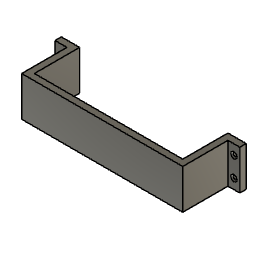
Bracket 185x155x50mm (Autodesk Fusion 360 design; units mm, degrees)
Autodesk Fusion 360 part; units mm, degrees
sketch "Outline" plane through (0, 0, 0) normal (0, 0, 1) x (1, 0, 0)
  line L0 (0, 0) -> (0, 56.9537) construction
  line L1 (0, 0) -> (93.5, 0)
  line L2 (93.5, 0) -> (93.5, 57)
  line L3 (93.5, 57) -> (116.5, 57)
  line L4 (116.5, 57) -> (116.5, 49)
  line L5 (-93.5, 57) -> (-116.5, 57)
  line L6 (-93.5, 0) -> (-93.5, 57)
  line L7 (0, 0) -> (-93.5, 0)
  line L8 (-101.5, -8) -> (-101.5, 49)
  line L9 (-101.5, 49) -> (-116.5, 49)
  line L10 (-116.5, 57) -> (-116.5, 49)
  line L11 (101.5, -8) -> (101.5, 49)
  line L12 (101.5, 49) -> (116.5, 49)
  line L13 (-101.5, -8) -> (101.5, -8)
  dimension "d2" = 187
  dimension "d3" = 57
  dimension "d6" = 23
  dimension "d8" = 8
  dimension "d9" = 8
  dimension "d10" = 8
  constraint coincident L0.start L1.start
  constraint vertical L0
  constraint perpendicular L0 L1
  constraint perpendicular L1 L2
  constraint perpendicular L2 L3
  constraint symmetric L0 L1.start L7.start
  constraint symmetric L0 L1.end L6.start
  constraint symmetric L0 L2.end L5.start
  constraint symmetric L0 L3.end L5.end
  constraint parallel L7 L13
  constraint vertical L8
  constraint horizontal L9
  constraint vertical L4
  constraint vertical L10
  measures "d2" distance of L1.end L6.start
  measures "d3" distance of L1.end L2.end
  measures "d6" distance of L5.start L5.end
  measures "d8" distance of L6 L8
  measures "d9" distance of L5 L9
  measures "d10" distance of L7 L13
extrude "Extrude1" add sketch "Outline" along normal blind 50
sketch "Holes for Mounting" plane through (0, 49, 0) normal (0, -1, 0) x (1, 0, 0)
  line L0 (-116.5, 0) -> (-101.5, 0)
  line L1 (-101.5, 0) -> (-101.5, 50)
  line L2 (-101.5, 50) -> (-116.5, 50)
  line L3 (-116.5, 50) -> (-116.5, 0)
  line L4 (101.5, 0) -> (116.5, 0)
  line L5 (116.5, 0) -> (116.5, 50)
  line L6 (116.5, 50) -> (101.5, 50)
  line L7 (101.5, 50) -> (101.5, 0)
  line L8 (0, 0) -> (0, 29.5518) construction
  line L9 (-109, 50) -> (-109, 0) construction
  circle A0 centre (-109, 12.5) radius 4
  line L10 (-116.5, 25) -> (-101.5, 25) construction
  circle A1 centre (-109, 37.5) radius 4
  circle A2 centre (109, 12.5) radius 4
  circle A3 centre (109, 37.5) radius 4
  dimension "d13" = 25
  dimension "d14" = 8
  constraint coincident L8.start origin
  constraint vertical L8
  constraint midpoint L2 L9.start
  constraint midpoint L0 L9.end
  constraint coincident L9 A0.centre
  constraint midpoint L3 L10.start
  constraint midpoint L1 L10.end
  constraint symmetric A0 L10 A1
  constraint symmetric L8 A0 A2
  constraint symmetric L8 A1 A3
  measures "d13" distance of A0.centre A1.centre
  measures "d14" diameter of A0
hole "Hole1" at (-109, 49, 12.5) at (-109, 49, 37.5) at (109, 49, 12.5) at (109, 49, 37.5) direction (0, 1, 0) diameter 4.5 depth 15 tip angle 118 countersink diameter 7.8 countersink angle 90
sketch "Make those holes 3d printable" plane through (0, 49, 0) normal (0, -1, 0) x (1, 0, 0)
  circle A0 centre (-109, 37.5) radius 2.25
  circle A1 centre (-109, 12.5) radius 2.25
  circle A2 centre (-109, 12.5) radius 3.9
  circle A3 centre (-109, 37.5) radius 3.9
  line L0 (-116.5, 0) -> (-101.5, 0)
  line L1 (-101.5, 0) -> (-101.5, 50)
  line L2 (-101.5, 50) -> (-116.5, 50)
  line L3 (-116.5, 50) -> (-116.5, 0)
  circle A4 centre (109, 12.5) radius 2.25
  circle A5 centre (109, 12.5) radius 3.9
  circle A6 centre (109, 37.5) radius 3.9
  line L4 (101.5, 0) -> (116.5, 0)
  line L5 (116.5, 0) -> (116.5, 50)
  line L6 (116.5, 50) -> (101.5, 50)
  line L7 (101.5, 50) -> (101.5, 0)
  circle A7 centre (109, 37.5) radius 2.25
  line L8 (0, 0) -> (0, 31.3528) construction
  line L9 (-109, 12.5) -> (-109, 37.5) construction
  line L10 (-109, 15.682) -> (-107.409, 14.091)
  line L11 (-109, 15.682) -> (-110.591, 14.091)
  line L12 (-109, 37.5) -> (-109, 47.9653) construction
  line L13 (-109, 40.682) -> (-107.409, 39.091)
  line L14 (-109, 40.682) -> (-110.591, 39.091)
  line L15 (109, 40.682) -> (110.591, 39.091)
  line L16 (109, 40.682) -> (107.409, 39.091)
  line L17 (109, 15.682) -> (110.591, 14.091)
  line L18 (109, 15.682) -> (107.409, 14.091)
  constraint coincident L8.start origin
  constraint vertical L8
  constraint coincident A1.centre A2.centre
  constraint coincident A0.centre A3.centre
  constraint coincident L9 L10.start
  constraint coincident A1 L10.end
  constraint tangent A1 L10
  constraint coincident A1 L11.end
  constraint tangent A1 L11
  constraint perpendicular L10 L11
  constraint parallel L9 L12
  constraint coincident L12 L13.start
  constraint coincident A0 L13.end
  constraint tangent A0 L13
  constraint coincident A0 L14.end
  constraint tangent A0 L14
  constraint perpendicular L13 L14
  constraint symmetric L8 L10.start L17.start
  constraint symmetric L8 L10.end L18.end
  constraint symmetric L8 L11.end L17.end
  constraint symmetric L8 L13.start L15.start
  constraint symmetric L8 L13.end L16.end
  constraint symmetric L8 L14.end L15.end
extrude "Extrude2" cut sketch "Make those holes 3d printable" against normal blind 8 contours A0 L13 L14 | A1 L10 L11 | A4 L17 L18 | A7 L15 L16
equation "d6 = 15 mm + 8 mm"
equation "d9 = d8"
equation "d10 = d8"
